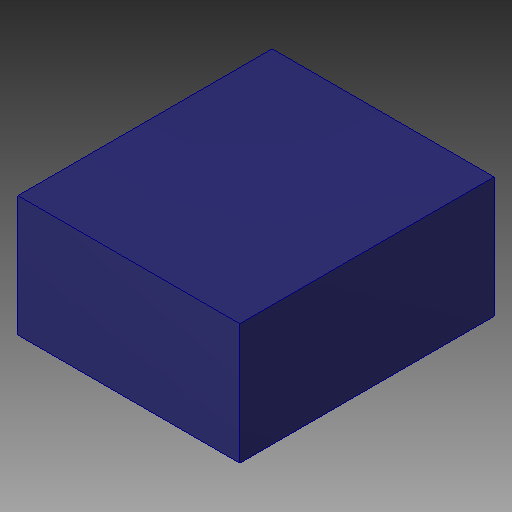
# Autodesk Inventor part: 3296W-1-103LF_11.550000
Saved by Autodesk Inventor 2019 (Build 230136000, 136)
## iProperties
Created: 2019-10-02
Part Number: 3296W-1-103LF_11.550000
Material: Generic
Document SubType Name: Modeling
Designer: rybit
Density: 1 g/cm^3
Appearance: SHDR3W54P0X254_1X3_953X483X115_11.550000, 3296W-1-103LF_11.550000
Author: rybit
Autodesk Inventor part; units mm, degrees
ref_plane "YZ Plane" through (0, 0, 0) normal (1, 0, 0) x (0, 1, 0)
ref_plane "XZ Plane" through (0, 0, 0) normal (0, 1, 0) x (-1, 0, 0)
ref_plane "XY Plane" through (0, 0, 0) normal (0, 0, 1) x (1, 0, 0)
sketch3d "SHDR3W54P0X254_1X3_953X483X115_11.550000, 3296W-1-103LF_11.5"
  constraints: 8 end point
sketch "SHDR3W54P0X254_1X3_953X483X115_11.550000, 3296W-1-103LF_11.550000_1" plane through (0, 0, 0) normal (0, 0, 1) x (1, 0, 0)
  line L0 (-7.585, 2.8) -> (2.495, 2.8)
  line L1 (2.495, 2.8) -> (2.495, -2.685)
  line L2 (2.495, -2.685) -> (-7.585, -2.685)
  line L3 (-7.585, -2.685) -> (-7.585, 2.8)
extrude "Extrusion1" add sketch "SHDR3W54P0X254_1X3_953X483X115_11.550000, 3296W-1-103LF_11.550000_1" along normal blind 11.55
body "Solid1"
